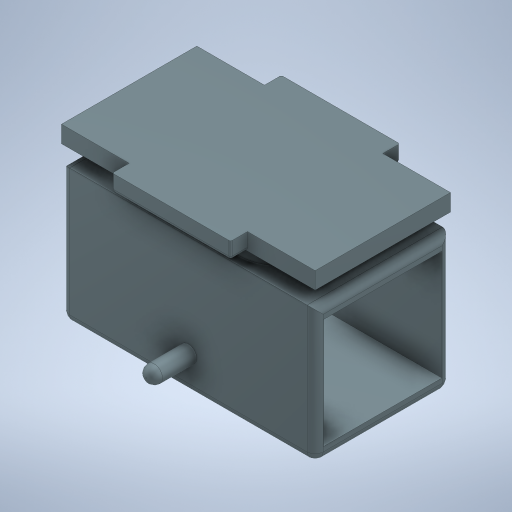
# Autodesk Inventor part: Battery Container
Saved by Autodesk Inventor 2023 (Build 270158000, 158)
## iProperties
Created: 2022-10-27
Part Number: Battery Container
Material: Iron, Malleable
Document SubType Name: Modeling
Designer: cheng
Density: 7.15 g/cm^3
Appearance: Lead
Mass: 3316.8 g
Surface Area: 1313.7 cm^2
Volume: 463.888 cm^3
Author: cheng
Autodesk Inventor part; units mm, degrees
ref_plane "YZ Plane" through (0, 0, 0) normal (1, 0, 0) x (0, 1, 0)
ref_plane "XZ Plane" through (0, 0, 0) normal (0, 1, 0) x (-1, 0, 0)
ref_plane "XY Plane" through (0, 0, 0) normal (0, 0, 1) x (1, 0, 0)
sketch "Sketch1" plane through (0, 0, 0) normal (0, 1, 0) x (-1, 0, 0)
  line L0 (75, -40) -> (-75, -40)
  line L1 (-75, -40) -> (-75, 40)
  line L2 (-75, 40) -> (75, 40)
  line L3 (75, 40) -> (75, -40)
  line L4 (75, -40) -> (-75, 40) construction
  line L5 (-75, -40) -> (75, 40) construction
  point P0 (0, 0)
  dimension "d0" = 80
  dimension "d1" = 150
  constraints: 12 end point, 2 midpoint, 2 parallel, 1 horizontal, 1 perpendicular
  measures "d0" distance of L0.end L1.end
  measures "d1" distance of L0.start L0.end
extrude "Extrusion1" add sketch "Sketch1" along normal blind 80
sketch "Sketch2" plane through (75, 0, 40) normal (1, 0, 0) x (0, 0, -1)
  line L0 (0, 0) -> (0, 80) projected
  line L1 (0, 40) -> (80, 40)
  line L2 (80, 0) -> (80, 80) projected
  line L3 (40, 0) -> (40, 80)
  line L4 (0, 80) -> (80, 80) projected
  line L5 (75, 72.5) -> (5, 72.5)
  line L6 (5, 72.5) -> (5, 7.5)
  line L7 (5, 7.5) -> (75, 7.5)
  line L8 (75, 7.5) -> (75, 72.5)
  line L9 (75, 72.5) -> (5, 7.5) construction
  line L10 (5, 72.5) -> (75, 7.5) construction
  point P0 (40, 40)
  dimension "d4" = 70
  dimension "d5" = 65
  constraints: 16 end point, 6 midpoint, 2 parallel, 1 horizontal, 1 perpendicular
  measures "d4" distance between parallel lines of L8 L6
  measures "d5" distance between parallel lines of L5 L7
extrude "Extrusion2" cut sketch "Sketch2" against normal blind 143.6625 contours L6 L5 L3 L1 | L1 L3 L7 L6 | L3 L5 L8 L1 | L1 L8 L7 L3
sketch "Sketch8" plane through (-75, 0, 40) normal (0, 0, 1) x (1, 0, 0)
  line L0 (0, 0) -> (0, 80) projected
  line L1 (0, 40) -> (75, 40) construction
  line L2 (75, 40) -> (75, 0) construction
  line L3 (0, 20) -> (75, 20) construction
  circle A0 centre (75, 20) radius 5
  dimension "d24" = 10
  constraints: 6 end point, 2 midpoint, 1 centre point, 1 coincident, 1 horizontal, 1 parallel, 1 perpendicular, 1 point on line
  measures "d24" diameter of A0
extrude "Extrusion5" add sketch "Sketch8" along normal blind 25
sketch "Sketch9" plane through (75, 0, -40) normal (0, 0, -1) x (-1, 0, 0)
  line L0 (0, 0) -> (0, 80) projected
  line L1 (0, 40) -> (75, 40) construction
  line L2 (75, 40) -> (75, 0) construction
  circle A0 centre (75, 20) radius 5 projected
  line L3 (0, 20) -> (75, 20) construction
  circle A1 centre (75, 20) radius 5
  dimension "d25" = 10
  constraints: 6 end point, 2 horizontal, 1 centre point, 1 coincident, 1 midpoint, 1 perpendicular, 1 point on line
  measures "d25" diameter of A1
extrude "Extrusion6" add sketch "Sketch9" along normal blind 25
fillet "Fillet1" radius 4.7625 1 edges at (-5, 20, 65)
fillet "Fillet2" radius 4.7625 1 edges at (5, 20, -65)
fillet "Fillet3" radius 4.7625 10 edges at (-75, 40, -40) (-75, 40, 40) (75, 40, 40) (75, 40, -40) (-75, 80, 0) (75, 80, 0) (-75, 0, 0) (0, 0, -40) (75, 0, 0) (0, 0, 40)
sketch "Sketch10" plane through (0, 80, 0) normal (0, 1, 0) x (1, 0, 0)
  line L0 (50, 35) -> (-50, 35)
  line L1 (-50, 35) -> (-50, -35)
  line L2 (-50, -35) -> (50, -35)
  line L3 (50, -35) -> (50, 35)
  line L4 (50, 35) -> (-50, -35) construction
  line L5 (-50, 35) -> (50, -35) construction
  line L6 (40, 25) -> (-40, 25)
  line L7 (-40, 25) -> (-40, -25)
  line L8 (-40, -25) -> (40, -25)
  line L9 (40, -25) -> (40, 25)
  line L10 (40, 25) -> (-40, -25) construction
  line L11 (-40, 25) -> (40, -25) construction
  point P0 (0, 0)
  dimension "d29" = 70
  dimension "d30" = 100
  dimension "d31" = 10
  dimension "d32" = 10
  constraints: 24 end point, 4 midpoint, 4 parallel, 2 horizontal, 2 perpendicular
  measures "d29" distance of L2.end L0.start
  measures "d30" distance of L0.start L0.end
  measures "d31" distance between parallel lines of L0 L6
  measures "d32" distance between parallel lines of L1 L7
extrude "Extrusion7" add sketch "Sketch10" along normal blind 10
sketch "Sketch11" plane through (0, 90, 0) normal (0, 1, 0) x (1, 0, 0)
  line L0 (75.0062, 40.005) -> (-75.0062, 40.005)
  line L1 (-75.0062, 40.005) -> (-75.0062, -40.005)
  line L2 (-75.0062, -40.005) -> (75.0062, -40.005)
  line L3 (75.0062, -40.005) -> (75.0062, 40.005)
  line L4 (75.0062, 40.005) -> (-75.0062, -40.005) construction
  line L5 (-75.0062, 40.005) -> (75.0062, -40.005) construction
  point P0 (0, 0)
  dimension "d35" = 80.01
  dimension "d36" = 150.0124
  constraints: 12 end point, 2 midpoint, 2 parallel, 1 horizontal, 1 perpendicular
  measures "d35" distance of L2.end L0.start
  measures "d36" distance of L0.start L0.end
extrude "Extrusion8" add sketch "Sketch11" along normal blind 10
sketch "Sketch12" plane through (-75.0062, 90, 40.005) normal (0, 0, 1) x (1, 0, 0)
  line L0 (150.0124, 10) -> (0, 10) construction
  line L1 (150.0124, 0) -> (0, 0) construction
  line L2 (0, 10) -> (150.0124, 0) construction
  line L3 (0, 0) -> (150.0124, 10) construction
  line L4 (35.0062, 0) -> (115.0062, 0) projected
  line L5 (110.0062, 10) -> (40.0062, 10)
  line L6 (40.0062, 10) -> (40.0062, 0)
  line L7 (40.0062, 0) -> (110.0062, 0)
  line L8 (110.0062, 0) -> (110.0062, 10)
  line L9 (110.0062, 10) -> (40.0062, 0) construction
  line L10 (40.0062, 10) -> (110.0062, 0) construction
  point P0 (75.0062, -90)
  point P1 (75.0062, 5)
  dimension "d39" = 70
  constraints: 16 end point, 3 midpoint, 2 parallel, 1 horizontal, 1 perpendicular, 1 point on line
  measures "d39" distance between parallel lines of L8 L6
extrude "Extrusion9" add sketch "Sketch12" along normal blind 10
sketch "Sketch13" plane through (75.0062, 90, -40.005) normal (0, 0, -1) x (-1, 0, 0)
  line L0 (0, 0) -> (150.0124, 0) projected
  line L1 (150.0124, 0) -> (150.0124, 10) projected
  line L2 (0, 10) -> (150.0124, 10) projected
  line L3 (0, 0) -> (0, 10) projected
  line L4 (0, 10) -> (150.0124, 0) construction
  line L5 (150.0124, 10) -> (0, 0) construction
  line L6 (35.0062, 0) -> (115.0062, 0) projected
  line L7 (110.0062, 10) -> (40.0062, 10)
  line L8 (40.0062, 10) -> (40.0062, 0)
  line L9 (40.0062, 0) -> (110.0062, 0)
  line L10 (110.0062, 0) -> (110.0062, 10)
  line L11 (110.0062, 10) -> (40.0062, 0) construction
  line L12 (40.0062, 10) -> (110.0062, 0) construction
  point P0 (75.0062, -90)
  point P1 (75.0062, 5)
  point P2 (110.0062, 10)
  point P3 (40.0062, 10)
  dimension "d42" = 70
  constraints: 16 end point, 3 midpoint, 2 parallel, 1 horizontal, 1 perpendicular, 1 point on line
  measures "d42" distance between parallel lines of L10 L8
extrude "Extrusion10" add sketch "Sketch13" along normal blind 10 contours L8 L2 L10 L0
fillet "Fillet4" radius 25.4 4 edges at (50, 85, -35) (50, 85, 35) (-50, 85, 35) (-50, 85, -35)
fillet "Fillet5" radius 1 4 edges at (35, 95, 50.005) (-35, 95, 50.005) (-35, 95, -50.005) (35, 95, -50.005)
fillet "Fillet7" radius 2 10 edges at (34.7071, 90, 49.7121) (35, 90, 44.505) (-34.7071, 90, 49.7121) (-35, 90, 44.505) (0, 90, 50.005) (-34.7071, 90, -49.7121) (-35, 90, -44.505) (34.7071, 90, -49.7121) (35, 90, -44.505) (0, 90, -50.005)
body "Solid1"
